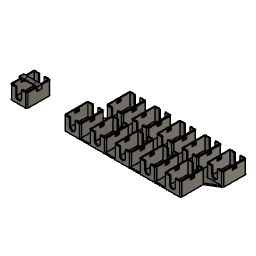
SolenoidHolder2 v13 (Autodesk Fusion 360 design; units mm, degrees)
Autodesk Fusion 360 part; units mm, degrees
sketch "BaseSketch" plane through (0, 0, 0) normal (0, 0, 1) x (1, 0, 0) in component "Box"
  line L0 (-15.2, 22.05) -> (15.2, 22.05)
  line L1 (15.2, 22.05) -> (15.2, -22.05)
  line L2 (15.2, -22.05) -> (-15.2, -22.05)
  line L3 (-15.2, -22.05) -> (-15.2, 22.05)
  line L4 (-15.2, 22.05) -> (15.2, -22.05) construction
  line L5 (15.2, 22.05) -> (-15.2, -22.05) construction
  dimension "d4" = 30.4
  dimension "d5" = 44.1
  constraint horizontal L0
  constraint perpendicular L0 L1
  constraint parallel L0 L2
  constraint parallel L1 L3
  constraint coincident L4 origin
  constraint coincident L5 origin
  measures "d4" distance of L1.end L2.end
  measures "d5" distance of L0 L2
extrude "ExtrudeBase" add sketch "BaseSketch" along normal blind 2.4 makes body 1 in component "Box"
sketch "SidesSketch" plane through (0, 0, 2.4) normal (0, 0, 1) x (-1, 0, 0) in component "Box"
  line L0 (15.2, 22.05) -> (-15.2, 22.05)
  line L1 (-15.2, 22.05) -> (-15.2, -22.05)
  line L2 (-15.2, -22.05) -> (15.2, -22.05)
  line L3 (15.2, -22.05) -> (15.2, 22.05)
  line L4 (13.2, -20.05) -> (-13.2, -20.05)
  line L5 (-13.2, -20.05) -> (-13.2, 20.05)
  line L6 (-13.2, 20.05) -> (13.2, 20.05)
  line L7 (13.2, 20.05) -> (13.2, -20.05)
  line L8 (13.2, -20.05) -> (-13.2, 20.05) construction
  line L9 (-13.2, -20.05) -> (13.2, 20.05) construction
  dimension "d9" = 26.4
  dimension "d10" = 40.1
  constraint horizontal L4
  constraint perpendicular L4 L5
  constraint parallel L4 L6
  constraint parallel L5 L7
  constraint coincident L8 origin
  constraint coincident L9 origin
  measures "d9" distance of L5.end L6.end
  measures "d10" distance of L4.end L5.end
extrude "ExtrudeEdgeOfBox" add sketch "SidesSketch" along normal blind 23.2 bodies 1 in component "Box"
sketch "TopSlotSketch" plane through (0, 22.05, 0) normal (0, 1, 0) x (-1, 0, 0) in component "Box"
  line L0 (-15.2, 0) -> (15.2, 0)
  line L1 (15.2, 0) -> (15.2, 25.6)
  line L2 (15.2, 25.6) -> (-15.2, 25.6)
  line L3 (-15.2, 25.6) -> (-15.2, 0)
  line L4 (0, 0) -> (0, -0.4112) construction
  line L5 (0, -0.4112) -> (0, 25.6) construction
  line L6 (-5.3, 25.6) -> (-5.3, 11)
  arc A0 (-5.3, 11) -> (5.3, 11) centre (0, 11) ccw
  line L7 (5.3, 11) -> (5.3, 25.6)
  arc A1 (5.3, 25.6) -> (-5.3, 25.6) centre (0, 25.6) ccw
  line L8 (0, 25.6) -> (0, 11) construction
  dimension "d19" = 10.6
  dimension "d49" = 11
  constraint coincident L4.start origin
  constraint perpendicular L0 L4
  constraint midpoint L2 L5.end
  constraint perpendicular L2 L5
  constraint tangent L6 A0
  constraint tangent A0 L7
  constraint parallel L6 L7
  constraint tangent L7 A1
  constraint tangent L6 A1
  constraint coincident L5 A0.centre
  constraint perpendicular L2 L8
  constraint coincident L5.end A1.centre
  measures "d19" diameter of A0
  measures "d49" distance of L4.start A0.centre
extrude "Extrude4" cut sketch "TopSlotSketch" against normal up to surface (44.1 mm away) contours L2 L6 A0 L7 bodies 1 in component "Box"
sketch "SideSlotsSketch" plane through (15.2, 0, 0) normal (1, 0, 0) x (0, 1, 0) in component "Box"
  line L0 (-22.05, 0) -> (22.05, 0)
  line L1 (22.05, 0) -> (22.05, 25.6)
  line L2 (22.05, 25.6) -> (-22.05, 25.6)
  line L3 (-22.05, 25.6) -> (-22.05, 0)
  line L4 (4, 23.2) -> (-4, 23.2)
  line L5 (-4, 23.2) -> (-4, 19.4)
  line L6 (-4, 19.4) -> (4, 19.4)
  line L7 (4, 19.4) -> (4, 23.2)
  line L8 (4, 23.2) -> (-4, 19.4) construction
  line L9 (-4, 23.2) -> (4, 19.4) construction
  point P0 (0, 21.3)
  dimension "d22" = 8
  dimension "d23" = 3.8
  dimension "d50" = 2.4
  constraint horizontal L4
  constraint perpendicular L4 L5
  constraint parallel L4 L6
  constraint parallel L5 L7
  constraint coincident L8 P0
  constraint coincident L9 P0
  constraint vertical origin P0
  measures "d22" distance of L5.end L6.end
  measures "d23" distance of L4.end L5.end
  measures "d50" distance of L2 L4
extrude "Extrude5" cut sketch "SideSlotsSketch" against normal up to surface (30.4 mm away) contours L4 L5 L6 L7 bodies 1 in component "Box"
sketch "HolderSketch" plane through (0, 0, 0) normal (0, 1, 0) x (1, 0, 0) in component "Holder"
  line L0 (-15.2, 0) -> (-15.2, -25.6)
  line L1 (-15.3, -25.8) -> (-15.3, -23.1)
  line L2 (-15.3, -23.1) -> (-14.3, -23.1)
  line L3 (-14.3, -23.1) -> (-16.1, -19.9823)
  line L4 (-16.1, -19.9823) -> (-16.9, -19.9823)
  line L5 (-16.9, -19.9823) -> (-16.9, -27.4)
  line L6 (-16.9, -27.4) -> (16.9, -27.4)
  line L7 (16.9, -27.4) -> (16.9, -19.9823)
  line L8 (16.9, -19.9823) -> (16.1, -19.9823)
  line L9 (16.1, -19.9823) -> (14.3, -23.1)
  line L10 (14.3, -23.1) -> (15.3, -23.1)
  line L11 (15.3, -23.1) -> (15.3, -25.8)
  line L12 (5.3, -25.6) -> (15.2, -25.6)
  line L13 (-15.2, 0) -> (-15.2, -25.6)
  line L14 (15.2, 0) -> (15.2, -25.6)
  line L15 (-13.2, -23.2) -> (-15.2, -23.2)
  line L16 (15.2, -19.4) -> (13.2, -19.4)
  line L17 (-13.2, -19.4) -> (-15.2, -19.4)
  line L18 (12.6, -25.8) -> (12.6, -23.4)
  line L19 (12.6, -23.4) -> (8.1, -23.4)
  line L20 (8.1, -23.4) -> (8.1, -25.8)
  line L21 (13.2, -2.4) -> (13.2, -25.6)
  line L22 (5.3, -25.6) -> (5.3, -11)
  line L23 (0, -1.75) -> (0, -22.5)
  line L24 (-8.1, -23.4) -> (-8.1, -25.8)
  line L25 (-12.6, -23.4) -> (-8.1, -23.4)
  line L26 (-12.6, -25.8) -> (-12.6, -23.4)
  line L27 (15.3, -25.8) -> (12.6, -25.8)
  line L28 (-12.6, -25.8) -> (-15.3, -25.8)
  line L29 (-8.1, -25.8) -> (-8.1, -26.4)
  line L30 (-8.1, -26.4) -> (8.1, -26.4)
  line L31 (8.1, -26.4) -> (8.1, -25.8)
  dimension "d30" = 0.2
  dimension "d31" = 0.1
  dimension "d32" = 0.1
  dimension "d33" = 0.1
  dimension "d35" = 1.6
  dimension "d36" = 1.6
  dimension "d37" = 1.6
  dimension "d38" = 1
  dimension "d40" = 1
  dimension "d51" = 0.6
  dimension "d52" = 2.8
  dimension "d53" = 2.2
  dimension "d55" = 0.6
  dimension "d56" = 60
  dimension "d58" = 60
  dimension "d59" = 0.8
  dimension "d60" = 0.8
  constraint parallel L0 L1
  constraint perpendicular L1 L2
  constraint perpendicular L1 L4
  constraint perpendicular L4 L5
  constraint perpendicular L5 L6
  constraint perpendicular L6 L7
  constraint perpendicular L5 L8
  constraint parallel L8 L10
  constraint perpendicular L10 L11
  constraint horizontal L27
  constraint collinear L2 L10
  constraint perpendicular L12 L18
  constraint perpendicular L18 L19
  constraint coincident L20.end L27
  constraint perpendicular L20 L27
  constraint symmetric L18.start L23 L26.start
  constraint symmetric L18.end L23 L25.start
  constraint symmetric L19.end L23 L24.start
  constraint symmetric L20.end L23 L24.end
  constraint perpendicular L23 L30
  constraint vertical L31
  constraint horizontal L28
  constraint vertical L29
  measures "d30" distance of L12 L27
  measures "d31" distance of L1 L13
  measures "d32" distance of L11 L14
  measures "d33" distance of L2 L15
  measures "d35" distance of L1 L5
  measures "d36" distance of L6 L27
  measures "d37" distance of L7 L11
  measures "d38" distance of L1.end L2.end
  measures "d40" distance of L9.end L10.end
  measures "d51" distance of L18 L21
  measures "d52" distance of L20 L22
  measures "d53" distance of L12 L19
  measures "d55" distance of L28 L30
  measures "d56" angle of L2 L3
  measures "d58" angle of L9 L10
  measures "d59" distance of L7.end L8.end
  measures "d60" distance of L3.end L4.end
extrude "Extrude2" add sketch "HolderSketch" along normal blind 3.975 and the other way blind 3.975 separate body contours L0 L2 L3 L13 | L0 L1 L2 L3 L4 L5 L6 L7 L8 L9 L10 L11 L12 L13 L14 L18 L20 L24 L25 L26 L27 L28 L29 L30 L31 | L9 L10 L14 | L12 L18 L19 L20 makes body 2 in component "Holder"
fillet "Fillet1" radius 2 4 edges at (15.2, 22.05, 12.8) (-15.2, 22.05, 12.8) (-15.2, -22.05, 12.8) (15.2, -22.05, 12.8) on bodies 1 in component "Box"
fillet "Fillet1" radius 0.6 6 edges at (15.2, 0, 25.6) (10.25, -22.05, 25.6) (-10.25, -22.05, 25.6) (-15.2, 0, 25.6) (-10.25, 22.05, 25.6) (10.25, 22.05, 25.6) on bodies 1 in component "Box"
copy_body "CopyPasteBodies1" bodies 1 makes body 3 in component "MultiFrame"
move_body "Move1" bodies 3 to x (1, 0, 0) y (0, 1, 0) z (0, 0, 1) at (100, 0, 0) in component "MultiFrame"
pattern_linear "R-Pattern1" count 5 spacing 46.6 along (1, 0, 0) count 2 spacing 55 along (0, 1, 0) of bodies 3 makes body 4 at (151.6667, -6.6833, 0) makes body 5 at (198.2667, -6.6833, 0) makes body 6 at (244.8667, -6.6833, 0) makes body 7 at (291.4667, -6.6833, 0) makes body 8 at (105.0667, 48.3167, 0) makes body 9 at (151.6667, 48.3167, 0) makes body 10 at (198.2667, 48.3167, 0) makes body 11 at (244.8667, 48.3167, 0) makes body 12 at (291.4667, 48.3167, 0) in component "MultiFrame"
move_body "Move2" bodies 8 12 10 9 11 to x (1, 0, 0) y (0, 1, 0) z (0, 0, 1) at (23.3, 0, 0) in component "MultiFrame"
sketch "Base" plane through (0, 0, 0) normal (0, 0, -1) x (1, 0, 0) in component "MultiFrame"
  arc A0 (86.8, 22.05) -> (84.8, 20.05) centre (86.8, 20.05) ccw
  line L0 (84.8, 20.05) -> (84.8, -20.05)
  arc A1 (84.8, -20.05) -> (86.8, -22.05) centre (86.8, -20.05) ccw
  line L1 (86.8, -22.05) -> (113.2, -22.05)
  arc A2 (113.2, -22.05) -> (115.2, -20.05) centre (113.2, -20.05) ccw
  line L2 (115.2, -20.05) -> (115.2, 20.05)
  arc A3 (115.2, 20.05) -> (113.2, 22.05) centre (113.2, 20.05) ccw
  line L3 (113.2, 22.05) -> (86.8, 22.05)
  line L4 (84.8, 20.05) -> (84.8, -20.05)
  arc A4 (84.8, -20.05) -> (86.8, -22.05) centre (86.8, -20.05) ccw
  line L5 (108.1, -34.95) -> (108.1, -75.05)
  line L6 (301.6, -20.05) -> (301.6, 20.05)
  arc A5 (324.9, -34.95) -> (322.9, -32.95) centre (322.9, -34.95) ccw
  line L7 (324.9, -75.05) -> (324.9, -34.95)
  arc A6 (322.9, -77.05) -> (324.9, -75.05) centre (322.9, -75.05) ccw
  line L8 (86.8, -22.05) -> (108.1, -34.95)
  line L9 (110.1, -77.05) -> (322.9, -77.05)
  line L10 (322.9, -32.95) -> (301.6, -20.05)
  line L11 (299.6, 22.05) -> (86.8, 22.05)
  arc A7 (108.1, -75.05) -> (110.1, -77.05) centre (110.1, -75.05) ccw
  arc A8 (86.8, 22.05) -> (84.8, 20.05) centre (86.8, 20.05) ccw
  arc A9 (301.6, 20.05) -> (299.6, 22.05) centre (299.6, 20.05) ccw
  line L12 (97.45, -28.5) -> (315.5523, -28.5) construction
  circle A10 centre (136.5012, -28.5) radius 1.4
  circle A11 centre (206.5012, -28.5) radius 1.4
  circle A12 centre (276.5012, -28.5) radius 1.4
  line L13 (138.5, -51) -> (138.5, -59) construction
  line L14 (154.7, -59) -> (154.7, -51) construction
  line L15 (138.5, -55) -> (154.7, -55) construction
  line L16 (185.1, -59) -> (185.1, -51) construction
  line L17 (201.3, -59) -> (201.3, -51) construction
  line L18 (185.1, -55) -> (201.3, -55) construction
  line L19 (231.7, -59) -> (231.7, -51) construction
  line L20 (247.9, -51) -> (247.9, -59) construction
  line L21 (231.7, -55) -> (247.9, -55) construction
  line L22 (278.3, -51) -> (278.3, -59) construction
  line L23 (294.5, -51) -> (294.5, -59) construction
  line L24 (278.3, -55) -> (294.5, -55) construction
  circle A13 centre (146.6, -55) radius 1.4
  circle A14 centre (193.2, -55) radius 1.4
  circle A15 centre (239.8, -55) radius 1.4
  circle A16 centre (286.4, -55) radius 1.4
  line L25 (131.4, 4) -> (131.4, -4) construction
  line L26 (115.2, 0) -> (131.4, 0) construction
  line L27 (161.8, 4) -> (161.8, -4) construction
  line L28 (178, -4) -> (178, 4) construction
  line L29 (161.8, 0) -> (178, 0) construction
  line L30 (208.4, 4) -> (208.4, -4) construction
  line L31 (224.6, -4) -> (224.6, 4) construction
  line L32 (208.4, 0) -> (224.6, 0) construction
  line L33 (255, 4) -> (255, -4) construction
  line L34 (271.2, -4) -> (271.2, 4) construction
  line L35 (255, 0) -> (271.2, 0) construction
  circle A17 centre (123.3, 0) radius 1.4
  circle A18 centre (169.9, 0) radius 1.4
  circle A19 centre (216.5, 0) radius 1.4
  circle A20 centre (263.1, 0) radius 1.4
  point P0 (86.8, 22.05)
  point P1 (110.1, -77.05)
  point P2 (299.6, 22.05)
  point P3 (206.5012, -28.5)
  point P4 (136.5012, -28.5)
  point P5 (276.5012, -28.5)
  point P6 (146.6, -55)
  dimension "d75" = 70
  dimension "d76" = 70
  dimension "d78" = 2.8
  dimension "d79" = 2.8
  dimension "d80" = 2.8
  dimension "d88" = 2.8
  dimension "d89" = 2.8
  dimension "d90" = 2.8
  dimension "d91" = 2.8
  dimension "d92" = 2.8
  dimension "d93" = 2.8
  dimension "d94" = 2.8
  dimension "d95" = 2.8
  constraint coincident A1.end L1.start
  constraint coincident L5.start L8.end
  constraint coincident P1 L9.start
  constraint coincident A6.start L9.end
  constraint coincident A5.end L10.start
  constraint coincident L6.start L10.end
  constraint coincident P2 L11.start
  constraint coincident P0 A0.start
  constraint midpoint L8 L12.start
  constraint coincident L10 L12.end
  constraint midpoint L12 P3
  constraint coincident L12 P4
  constraint coincident L12 P5
  constraint coincident P4 A10.centre
  constraint coincident P3 A11.centre
  constraint coincident P5 A12.centre
  constraint horizontal L12
  constraint midpoint L13 L15.start
  constraint midpoint L14 L15.end
  constraint midpoint L15 P6
  constraint midpoint L16 L18.start
  constraint midpoint L17 L18.end
  constraint midpoint L19 L21.start
  constraint midpoint L20 L21.end
  constraint midpoint L22 L24.start
  constraint midpoint L23 L24.end
  constraint coincident P6 A13.centre
  constraint midpoint L18 A14.centre
  constraint midpoint L21 A15.centre
  constraint midpoint L24 A16.centre
  constraint midpoint L2 L26.start
  constraint midpoint L25 L26.end
  constraint midpoint L27 L29.start
  constraint midpoint L28 L29.end
  constraint midpoint L30 L32.start
  constraint midpoint L31 L32.end
  constraint midpoint L33 L35.start
  constraint midpoint L34 L35.end
  constraint midpoint L26 A17.centre
  constraint midpoint L29 A18.centre
  constraint midpoint L32 A19.centre
  constraint midpoint L35 A20.centre
  measures "d75" distance of P3 P4
  measures "d76" distance of P3 P5
  measures "d78" diameter of A10
  measures "d79" diameter of A11
  measures "d80" diameter of A12
  measures "d88" diameter of A13
  measures "d89" diameter of A14
  measures "d90" diameter of A15
  measures "d91" diameter of A16
  measures "d92" diameter of A17
  measures "d93" diameter of A18
  measures "d94" diameter of A19
  measures "d95" diameter of A20
extrude "ExtrudeBase'" add sketch "Base" against normal blind 2.4 contours L1 A2 L2 A3 L5 L6 A5 L7 A6 L8 L9 L10 L11 A7 A9 | A10 | A11 | A12 | A13 | A14 | A15 | A16 | A17 | A18 | A19 | A20 bodies 4 3 5 6 7 8 9 10 11 12 in component "MultiFrame"
extrude "CutScrewHoles" cut sketch "Base" against normal up to surface (2.4 mm away) contours A10 | A11 | A12 | A13 | A14 | A15 | A16 | A17 | A18 | A19 | A20 bodies 4 in component "MultiFrame"
component "Holder" placed x (1, 0, 0) y (0, 1, 0) z (0, 0, 1) at (0, 0, 0)
component "Box" placed x (1, 0, 0) y (0, 1, 0) z (0, 0, 1) at (0, 0, 0)
component "MultiFrame" placed x (1, 0, 0) y (0, 1, 0) z (0, 0, 1) at (0, 0, 0)
equation "solenoid_width = 26.4 mm"
equation "solenoid_height = 40.1 mm"
equation "case_edge = 2 mm"
equation "d4 = solenoid_width + 2 * case_edge"
equation "d5 = solenoid_height + 2 * case_edge"
equation "base_thickness = 2.4 mm"
equation "d7 = base_thickness"
equation "d9 = solenoid_width"
equation "d10 = solenoid_height"
equation "solenoid_depth = 23.2 mm"
equation "d12 = solenoid_depth"
equation "d22 = slot_width"
equation "d23 = slot_height"
equation "slot_width = 8 mm"
equation "slot_height = 3.8 mm"
equation "horiz_tab_slop = 0.1 mm"
equation "vert_tab_slop = 0.2 mm"
equation "d30 = vert_tab_slop"
equation "d31 = horiz_tab_slop"
equation "d32 = horiz_tab_slop"
equation "d33 = horiz_tab_slop"
equation "holder_thickness = 1.6 mm"
equation "d35 = holder_thickness"
equation "d36 = holder_thickness"
equation "d37 = holder_thickness"
equation "d38 = tab_insert_amount"
equation "tab_insert_amount = 1.0 mm"
equation "d40 = tab_insert_amount"
equation "tab_length_spacing = 0.2 mm"
equation "holder_width_gap = 0.05 mm"
equation "tab_angle = 60 deg"
equation "d58 = tab_angle"
equation "d61 = slot_width / 2 - ( holder_width_gap / 2 )"
equation "d63 = slot_width / 2 - ( holder_width_gap / 2 )"
equation "d71 = horizontal_spacing"
equation "d72 = vertical_spacing"
equation "d73 = -base_thickness"
equation "screw_diam = 2.8 mm"
equation "d78 = screw_diam"
equation "d79 = screw_diam"
equation "d80 = screw_diam"
equation "horizontal_spacing = 46.6 mm"
equation "vertical_spacing = 55 mm"
equation "d85 = horizontal_spacing / 2"
equation "d88 = screw_diam"
equation "d89 = screw_diam"
equation "d90 = screw_diam"
equation "d91 = screw_diam"
equation "d92 = screw_diam"
equation "d93 = screw_diam"
equation "d94 = screw_diam"
equation "d95 = screw_diam"
named bodies: "Box", "Holder", "MultiFrame", "Box (2)", "Box (3)", "Box (4)", "Box (5)", "Box (6)", "Box (7)", "Box (8)", "Box (9)"
